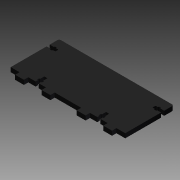
# Autodesk Inventor part: frontal base reforç
Saved by Autodesk Inventor 2012 SP1 (Build 160190100, 190)
## iProperties
Created: 2015-03-30
Part Number: frontal base reforç
Material: Default
Document SubType Name: Modeling
Designer: sheina
Density: 1 g/cm^3
Author: sheina
Autodesk Inventor part; units mm, degrees
ref_plane "YZ Plane" through (0, 0, 0) normal (1, 0, 0) x (0, 1, 0)
ref_plane "XZ Plane" through (0, 0, 0) normal (0, 1, 0) x (-1, 0, 0)
ref_plane "XY Plane" through (0, 0, 0) normal (0, 0, 1) x (1, 0, 0)
sketch "Boceto1" plane through (0, 0, 0) normal (0, 0, 1) x (1, 0, 0)
  line L0 (130, 10) -> (130, 65)
  line L1 (0, 65) -> (0, 10)
  line L2 (20, 10) -> (20, 5)
  line L3 (10, 5) -> (10, 10)
  line L4 (50, 10) -> (50, 5)
  line L5 (40, 5) -> (40, 10)
  line L6 (90, 10) -> (90, 5)
  line L7 (80, 5) -> (80, 10)
  line L8 (120, 10) -> (120, 5)
  line L9 (110, 5) -> (110, 10)
  line L10 (20, 5) -> (10, 5)
  line L11 (50, 5) -> (40, 5)
  line L12 (0, 10) -> (10, 10)
  line L13 (20, 10) -> (40, 10)
  line L14 (120, 5) -> (110, 5)
  line L15 (90, 5) -> (80, 5)
  line L16 (50, 10) -> (80, 10)
  line L17 (90, 10) -> (110, 10)
  line L18 (120, 10) -> (130, 10)
  line L19 (130, 65) -> (0, 65)
  point P0 (0, 0)
  dimension "d4" = 130
  dimension "d5" = 10
  dimension "d6" = 10
  dimension "d7" = 10
  dimension "d8" = 10
  dimension "d9" = 10
  dimension "d10" = 10
  dimension "d11" = 20
  dimension "d12" = 20
  dimension "d20" = 55
  constraints: 40 end point, 9 perpendicular, 6 parallel, 5 horizontal
  measures "d4" distance between parallel lines of L0 L1
  measures "d5" distance between parallel lines of L3 L2
  measures "d6" distance between parallel lines of L4 L5
  measures "d7" distance between parallel lines of L6 L7
  measures "d8" distance between parallel lines of L9 L8
  measures "d9" distance between parallel lines of L3 L1
  measures "d10" distance between parallel lines of L0 L8
  measures "d11" distance between parallel lines of L6 L9
  measures "d12" distance between parallel lines of L5 L2
  measures "d20" distance between parallel lines of L19 L13
extrude "Extrusión1" add sketch "Boceto1" along normal blind 5
fillet "Empalme1" radius 2 2 edges at (0, 65, 2.5) (130, 65, 2.5)
sketch "Boceto3" plane through (0, 0, 0) normal (0, 0, -1) x (-1, 0, 0)
  line L0 (-115.7878, 40.9736) -> (-8.9473, 40.9736) construction
  line L1 (-8.9473, 40.9736) -> (-8.9473, 10.5521) construction
  line L2 (-8.9473, 10.5521) -> (-115.7878, 10.5521) construction
  line L3 (-115.7878, 10.5521) -> (-115.7878, 40.9736) construction
  spline S0 degree 2 poles (-104.1512, 31.8359) (-104.5888, 31.8359) (-105.4543, 31.6219) (-105.8724, 31.4566) knots 0 0 0 1 2 2 2
  spline S1 degree 2 poles (-105.8724, 31.4566) (-106.2614, 31.2913) (-106.8351, 30.9412) (-107.0588, 30.7856) knots 0 0 0 1 2 2 2
  line L4 (-107.0588, 30.7856) -> (-107.156, 30.7856)
  line L5 (-107.156, 30.7856) -> (-107.156, 32.4874)
  spline S2 degree 2 poles (-107.156, 32.4874) (-106.6309, 32.7694) (-104.8319, 33.2265) (-104.0248, 33.2265) knots 0 0 0 1 2 2 2
  spline S3 degree 2 poles (-104.0248, 33.2265) (-103.2079, 33.2265) (-101.9923, 32.8958) (-101.4964, 32.5458) knots 0 0 0 1 2 2 2
  spline S4 degree 2 poles (-101.4964, 32.5458) (-100.9713, 32.1665) (-100.4267, 31.0676) (-100.4267, 30.3286) knots 0 0 0 1 2 2 2
  spline S5 degree 2 poles (-100.4267, 30.3286) (-100.4267, 29.3367) (-101.7298, 27.8391) (-102.6439, 27.6446) knots 0 0 0 1 2 2 2
  line L6 (-102.6439, 27.6446) -> (-102.6439, 27.5279)
  spline S6 degree 2 poles (-102.6439, 27.5279) (-102.2646, 27.4501) (-101.3992, 27.1001) (-101.0296, 26.75) knots 0 0 0 1 2 2 2
  spline S7 degree 2 poles (-101.0296, 26.75) (-100.6601, 26.4096) (-100.1933, 25.3205) (-100.1933, 24.5328) knots 0 0 0 1 2 2 2
  spline S8 degree 2 poles (-100.1933, 24.5328) (-100.1933, 23.7257) (-100.7476, 22.3545) (-101.2533, 21.8294) knots 0 0 0 1 2 2 2
  spline S9 degree 2 poles (-101.2533, 21.8294) (-101.7784, 21.2848) (-103.2663, 20.7208) (-104.2095, 20.7208) knots 0 0 0 1 2 2 2
  spline S10 degree 2 poles (-104.2095, 20.7208) (-105.1139, 20.7208) (-106.8838, 21.1584) (-107.4867, 21.4599) knots 0 0 0 1 2 2 2
  line L7 (-107.4867, 21.4599) -> (-107.4867, 23.1616)
  line L8 (-107.4867, 23.1616) -> (-107.37, 23.1616)
  spline S11 degree 2 poles (-107.37, 23.1616) (-106.8643, 22.7921) (-105.1528, 22.1114) (-104.3068, 22.1114) knots 0 0 0 1 2 2 2
  spline S12 degree 2 poles (-104.3068, 22.1114) (-103.8108, 22.1114) (-102.8189, 22.4226) (-102.4883, 22.7824) knots 0 0 0 1 2 2 2
  spline S13 degree 2 poles (-102.4883, 22.7824) (-102.1674, 23.1422) (-101.827, 23.9979) (-101.827, 24.6495) knots 0 0 0 1 2 2 2
  spline S14 degree 2 poles (-101.827, 24.6495) (-101.827, 25.301) (-102.2063, 26.1471) (-102.5466, 26.3902) knots 0 0 0 1 2 2 2
  spline S15 degree 2 poles (-102.5466, 26.3902) (-102.887, 26.6333) (-103.8108, 26.818) (-104.3554, 26.818) knots 0 0 0 1 2 2 2
  line L9 (-104.3554, 26.818) -> (-105.0361, 26.818)
  line L10 (-105.0361, 26.818) -> (-105.0361, 28.1503)
  line L11 (-105.0361, 28.1503) -> (-104.5013, 28.1503)
  spline S16 degree 2 poles (-104.5013, 28.1503) (-103.4218, 28.1503) (-102.0604, 29.1811) (-102.0604, 30.1633) knots 0 0 0 1 2 2 2
  spline S17 degree 2 poles (-102.0604, 30.1633) (-102.0604, 30.6203) (-102.4105, 31.2719) (-102.6925, 31.4663) knots 0 0 0 1 2 2 2
  spline S18 degree 2 poles (-102.6925, 31.4663) (-102.994, 31.6706) (-103.733, 31.8359) (-104.1512, 31.8359) knots 0 0 0 1 2 2 2
  spline S19 degree 2 poles (-88.5823, 26.9639) (-88.5823, 25.3205) (-89.9146, 22.6754) (-91.0329, 21.9364) knots 0 0 0 1 2 2 2
  spline S20 degree 2 poles (-91.0329, 21.9364) (-91.947, 21.3626) (-93.8238, 20.9736) (-95.2825, 20.9736) knots 0 0 0 1 2 2 2
  line L12 (-95.2825, 20.9736) -> (-98.0442, 20.9736)
  line L13 (-98.0442, 20.9736) -> (-98.0442, 32.9736)
  line L14 (-98.0442, 32.9736) -> (-95.3116, 32.9736)
  spline S21 degree 2 poles (-95.3116, 32.9736) (-93.6196, 32.9736) (-91.6941, 32.468) (-91.0134, 32.0206) knots 0 0 0 1 2 2 2
  spline S22 degree 2 poles (-91.0134, 32.0206) (-89.8562, 31.2524) (-88.5823, 28.7143) (-88.5823, 26.9639) knots 0 0 0 1 2 2 2
  spline S23 degree 2 poles (-90.2452, 26.9834) (-90.2452, 28.3642) (-91.1593, 30.3189) (-92.0637, 30.8731) knots 0 0 0 1 2 2 2
  spline S24 degree 2 poles (-92.0637, 30.8731) (-92.7055, 31.2524) (-94.1544, 31.5928) (-95.2338, 31.5928) knots 0 0 0 1 2 2 2
  line L15 (-95.2338, 31.5928) -> (-96.4494, 31.5928)
  line L16 (-96.4494, 31.5928) -> (-96.4494, 22.3545)
  line L17 (-96.4494, 22.3545) -> (-95.2338, 22.3545)
  spline S25 degree 2 poles (-95.2338, 22.3545) (-94.1739, 22.3545) (-92.5693, 22.6949) (-91.9178, 23.1519) knots 0 0 0 1 2 2 2
  spline S26 degree 2 poles (-91.9178, 23.1519) (-91.0815, 23.7159) (-90.2452, 25.583) (-90.2452, 26.9834) knots 0 0 0 1 2 2 2
  spline S27 degree 2 poles (-72.1431, 27.959) (-72.1431, 27.3107) (-72.605, 26.1438) (-73.0183, 25.7386) knots 0 0 0 1 2 2 2
  spline S28 degree 2 poles (-73.0183, 25.7386) (-73.5369, 25.2281) (-74.9389, 24.7013) (-76.0086, 24.7013) knots 0 0 0 1 2 2 2
  line L18 (-76.0086, 24.7013) -> (-77.135, 24.7013)
  line L19 (-77.135, 24.7013) -> (-77.135, 20.9736)
  line L20 (-77.135, 20.9736) -> (-78.464, 20.9736)
  line L21 (-78.464, 20.9736) -> (-78.464, 30.9736)
  line L22 (-78.464, 30.9736) -> (-75.9518, 30.9736)
  spline S29 degree 2 poles (-75.9518, 30.9736) (-75.0604, 30.9736) (-73.8124, 30.6819) (-73.3343, 30.3496) knots 0 0 0 1 2 2 2
  spline S30 degree 2 poles (-73.3343, 30.3496) (-72.7752, 29.9688) (-72.1431, 28.7937) (-72.1431, 27.959) knots 0 0 0 1 2 2 2
  spline S31 degree 2 poles (-73.5288, 27.9185) (-73.5288, 28.4372) (-73.8854, 29.1989) (-74.25, 29.442) knots 0 0 0 1 2 2 2
  spline S32 degree 2 poles (-74.25, 29.442) (-74.5661, 29.6527) (-75.4089, 29.8229) (-76.0329, 29.8229) knots 0 0 0 1 2 2 2
  line L23 (-76.0329, 29.8229) -> (-77.135, 29.8229)
  line L24 (-77.135, 29.8229) -> (-77.135, 25.8359)
  line L25 (-77.135, 25.8359) -> (-76.2274, 25.8359)
  spline S33 degree 2 poles (-76.2274, 25.8359) (-75.417, 25.8359) (-74.4202, 26.0952) (-74.0961, 26.4355) knots 0 0 0 1 2 2 2
  spline S34 degree 2 poles (-74.0961, 26.4355) (-73.7962, 26.7354) (-73.5288, 27.4404) (-73.5288, 27.9185) knots 0 0 0 1 2 2 2
  line L26 (-63.1398, 20.9736) -> (-64.8659, 20.9736)
  line L27 (-64.8659, 20.9736) -> (-68.0264, 24.9526)
  line L28 (-68.0264, 24.9526) -> (-69.5499, 24.9526)
  line L29 (-69.5499, 24.9526) -> (-69.5499, 20.9736)
  line L30 (-69.5499, 20.9736) -> (-70.8789, 20.9736)
  line L31 (-70.8789, 20.9736) -> (-70.8789, 30.9736)
  line L32 (-70.8789, 30.9736) -> (-68.3019, 30.9736)
  spline S35 degree 2 poles (-68.3019, 30.9736) (-67.4429, 30.9736) (-66.2841, 30.7872) (-65.7573, 30.4469) knots 0 0 0 1 2 2 2
  spline S36 degree 2 poles (-65.7573, 30.4469) (-65.2306, 30.1065) (-64.6228, 29.0449) (-64.6228, 28.2589) knots 0 0 0 1 2 2 2
  spline S37 degree 2 poles (-64.6228, 28.2589) (-64.6228, 27.1649) (-65.7411, 25.6819) (-66.6974, 25.3253) knots 0 0 0 1 2 2 2
  line L33 (-66.6974, 25.3253) -> (-63.1398, 20.9736)
  spline S38 degree 2 poles (-66.0086, 28.1535) (-66.0086, 28.5911) (-66.3165, 29.2637) (-66.6406, 29.4825) knots 0 0 0 1 2 2 2
  spline S39 degree 2 poles (-66.6406, 29.4825) (-66.9243, 29.6689) (-67.6779, 29.8229) (-68.229, 29.8229) knots 0 0 0 1 2 2 2
  line L34 (-68.229, 29.8229) -> (-69.5499, 29.8229)
  line L35 (-69.5499, 29.8229) -> (-69.5499, 26.0628)
  line L36 (-69.5499, 26.0628) -> (-68.3829, 26.0628)
  spline S40 degree 2 poles (-68.3829, 26.0628) (-67.8076, 26.0628) (-66.8919, 26.2654) (-66.5758, 26.5814) knots 0 0 0 1 2 2 2
  spline S41 degree 2 poles (-66.5758, 26.5814) (-66.2841, 26.8569) (-66.0086, 27.6349) (-66.0086, 28.1535) knots 0 0 0 1 2 2 2
  line L37 (-58.8611, 20.9736) -> (-62.7346, 20.9736)
  line L38 (-62.7346, 20.9736) -> (-62.7346, 21.9947)
  line L39 (-62.7346, 21.9947) -> (-61.4624, 21.9947)
  line L40 (-61.4624, 21.9947) -> (-61.4624, 29.9526)
  line L41 (-61.4624, 29.9526) -> (-62.7346, 29.9526)
  line L42 (-62.7346, 29.9526) -> (-62.7346, 30.9736)
  line L43 (-62.7346, 30.9736) -> (-58.8611, 30.9736)
  line L44 (-58.8611, 30.9736) -> (-58.8611, 29.9526)
  line L45 (-58.8611, 29.9526) -> (-60.1334, 29.9526)
  line L46 (-60.1334, 29.9526) -> (-60.1334, 21.9947)
  line L47 (-60.1334, 21.9947) -> (-58.8611, 21.9947)
  line L48 (-58.8611, 21.9947) -> (-58.8611, 20.9736)
  line L49 (-50.0604, 20.9736) -> (-51.5515, 20.9736)
  line L50 (-51.5515, 20.9736) -> (-55.9761, 29.596)
  line L51 (-55.9761, 29.596) -> (-55.9761, 20.9736)
  line L52 (-55.9761, 20.9736) -> (-57.216, 20.9736)
  line L53 (-57.216, 20.9736) -> (-57.216, 30.9736)
  line L54 (-57.216, 30.9736) -> (-55.3278, 30.9736)
  line L55 (-55.3278, 30.9736) -> (-51.3003, 23.0563)
  line L56 (-51.3003, 23.0563) -> (-51.3003, 30.9736)
  line L57 (-51.3003, 30.9736) -> (-50.0604, 30.9736)
  line L58 (-50.0604, 30.9736) -> (-50.0604, 20.9736)
  line L59 (-45.7006, 20.9736) -> (-45.7006, 29.7905)
  line L60 (-45.7006, 29.7905) -> (-49.0556, 29.7905)
  line L61 (-49.0556, 29.7905) -> (-49.0556, 30.9736)
  line L62 (-49.0556, 30.9736) -> (-41.0167, 30.9736)
  line L63 (-41.0167, 30.9736) -> (-41.0167, 29.7905)
  line L64 (-41.0167, 29.7905) -> (-44.3716, 29.7905)
  line L65 (-44.3716, 29.7905) -> (-44.3716, 20.9736)
  line L66 (-44.3716, 20.9736) -> (-45.7006, 20.9736)
  spline S42 degree 2 poles (-36.0977, 20.7954) (-37.0701, 20.7954) (-38.7152, 21.4518) (-39.3149, 22.1082) knots 0 0 0 1 2 2 2
  spline S43 degree 2 poles (-39.3149, 22.1082) (-39.9145, 22.7565) (-40.571, 24.7013) (-40.571, 25.9655) knots 0 0 0 1 2 2 2
  spline S44 degree 2 poles (-40.571, 25.9655) (-40.571, 27.2216) (-39.9308, 29.0855) (-39.323, 29.7743) knots 0 0 0 1 2 2 2
  spline S45 degree 2 poles (-39.323, 29.7743) (-38.7233, 30.4469) (-37.0863, 31.1519) (-36.0734, 31.1519) knots 0 0 0 1 2 2 2
  spline S46 degree 2 poles (-36.0734, 31.1519) (-35.571, 31.1519) (-34.6876, 31.006) (-34.3149, 30.8926) knots 0 0 0 1 2 2 2
  spline S47 degree 2 poles (-34.3149, 30.8926) (-33.9907, 30.7872) (-33.3181, 30.4874) (-32.9859, 30.3091) knots 0 0 0 1 2 2 2
  line L67 (-32.9859, 30.3091) -> (-32.9859, 28.7046)
  line L68 (-32.9859, 28.7046) -> (-33.0912, 28.7046)
  spline S48 degree 2 poles (-33.0912, 28.7046) (-33.2695, 28.8667) (-33.8205, 29.3205) (-34.2176, 29.5393) knots 0 0 0 1 2 2 2
  spline S49 degree 2 poles (-34.2176, 29.5393) (-34.5985, 29.75) (-35.498, 30.0174) (-36.0815, 30.0174) knots 0 0 0 1 2 2 2
  spline S50 degree 2 poles (-36.0815, 30.0174) (-36.7217, 30.0174) (-37.8643, 29.4907) (-38.2938, 28.9882) knots 0 0 0 1 2 2 2
  spline S51 degree 2 poles (-38.2938, 28.9882) (-38.7152, 28.4777) (-39.1852, 26.9299) (-39.1852, 25.9655) knots 0 0 0 1 2 2 2
  spline S52 degree 2 poles (-39.1852, 25.9655) (-39.1852, 24.9364) (-38.6909, 23.4534) (-38.2614, 22.9428) knots 0 0 0 1 2 2 2
  spline S53 degree 2 poles (-38.2614, 22.9428) (-37.84, 22.4485) (-36.7136, 21.9461) (-36.0815, 21.9461) knots 0 0 0 1 2 2 2
  spline S54 degree 2 poles (-36.0815, 21.9461) (-35.5061, 21.9461) (-34.5256, 22.2297) (-34.1447, 22.4404) knots 0 0 0 1 2 2 2
  spline S55 degree 2 poles (-34.1447, 22.4404) (-33.78, 22.6511) (-33.2371, 23.0887) (-33.0831, 23.2427) knots 0 0 0 1 2 2 2
  line L69 (-33.0831, 23.2427) -> (-32.9859, 23.2427)
  line L70 (-32.9859, 23.2427) -> (-32.9859, 21.6543)
  spline S56 degree 2 poles (-32.9859, 21.6543) (-33.3181, 21.5004) (-33.9016, 21.2167) (-34.3149, 21.0871) knots 0 0 0 1 2 2 2
  spline S57 degree 2 poles (-34.3149, 21.0871) (-34.7525, 20.9412) (-35.498, 20.7954) (-36.0977, 20.7954) knots 0 0 0 1 2 2 2
  line L71 (-32.8238, 20.9736) -> (-29.4526, 30.9736)
  line L72 (-29.4526, 30.9736) -> (-27.8157, 30.9736)
  line L73 (-27.8157, 30.9736) -> (-24.4445, 20.9736)
  line L74 (-24.4445, 20.9736) -> (-25.8465, 20.9736)
  line L75 (-25.8465, 20.9736) -> (-26.7541, 23.7694)
  line L76 (-26.7541, 23.7694) -> (-30.571, 23.7694)
  line L77 (-30.571, 23.7694) -> (-31.4786, 20.9736)
  line L78 (-31.4786, 20.9736) -> (-32.8238, 20.9736)
  line L79 (-27.1188, 24.9039) -> (-28.6666, 29.6122)
  line L80 (-28.6666, 29.6122) -> (-30.2063, 24.9039)
  line L81 (-30.2063, 24.9039) -> (-27.1188, 24.9039)
  line L82 (-21.1625, 20.9736) -> (-21.1625, 29.7905)
  line L83 (-21.1625, 29.7905) -> (-24.5175, 29.7905)
  line L84 (-24.5175, 29.7905) -> (-24.5175, 30.9736)
  line L85 (-24.5175, 30.9736) -> (-16.4786, 30.9736)
  line L86 (-16.4786, 30.9736) -> (-16.4786, 29.7905)
  line L87 (-16.4786, 29.7905) -> (-19.8335, 29.7905)
  line L88 (-19.8335, 29.7905) -> (-19.8335, 20.9736)
  line L89 (-19.8335, 20.9736) -> (-21.1625, 20.9736)
  constraints: 2 other
extrude "Extrusión3" cut sketch "Boceto3" against normal blind 1
sketch "Boceto4" plane through (0, 0, 0) normal (0, 0, -1) x (-1, 0, 0)
  line L0 (-31.7524, 12.5727) -> (-32.7524, 12.5727)
  line L1 (-31.7524, 9.7986) -> (-31.7524, 12.5727)
  line L2 (-31.7524, 14.9727) -> (-31.7524, 19.884)
  line L3 (-27.2524, 14.9727) -> (-27.2524, 12.5727)
  line L4 (-28.2524, 14.9727) -> (-27.2524, 14.9727)
  line L5 (-31.7524, 19.884) -> (-28.2524, 19.884)
  line L6 (-28.2524, 19.884) -> (-28.2524, 14.9727)
  line L7 (-27.2524, 12.5727) -> (-28.2524, 12.5727)
  line L8 (-28.2524, 12.5727) -> (-28.2524, 9.7986)
  line L9 (-32.7524, 12.5727) -> (-32.7524, 14.9727)
  line L10 (-32.7524, 14.9727) -> (-31.7524, 14.9727)
  line L11 (-31.7524, 9.7986) -> (-28.2524, 9.7986)
  line L12 (-101.7513, 12.6989) -> (-102.7513, 12.6989)
  line L13 (-101.7513, 9.9249) -> (-101.7513, 12.6989)
  line L14 (-101.7513, 15.0989) -> (-101.7513, 20.0103)
  line L15 (-97.2513, 15.0989) -> (-97.2513, 12.6989)
  line L16 (-98.2513, 15.0989) -> (-97.2513, 15.0989)
  line L17 (-101.7513, 20.0103) -> (-98.2513, 20.0103)
  line L18 (-98.2513, 20.0103) -> (-98.2513, 15.0989)
  line L19 (-97.2513, 12.6989) -> (-98.2513, 12.6989)
  line L20 (-98.2513, 12.6989) -> (-98.2513, 9.9249)
  line L21 (-102.7513, 12.6989) -> (-102.7513, 15.0989)
  line L22 (-102.7513, 15.0989) -> (-101.7513, 15.0989)
  line L23 (-101.7513, 9.9249) -> (-98.2513, 9.9249)
  line L24 (-123.0301, 50.7481) -> (-123.0301, 49.7481)
  line L25 (-120.2561, 50.7481) -> (-123.0301, 50.7481)
  line L26 (-125.4301, 50.7481) -> (-130.3414, 50.7481)
  line L27 (-125.4301, 55.2481) -> (-123.0301, 55.2481)
  line L28 (-125.4301, 54.2481) -> (-125.4301, 55.2481)
  line L29 (-130.3414, 50.7481) -> (-130.3414, 54.2481)
  line L30 (-130.3414, 54.2481) -> (-125.4301, 54.2481)
  line L31 (-123.0301, 55.2481) -> (-123.0301, 54.2481)
  line L32 (-123.0301, 54.2481) -> (-120.2561, 54.2481)
  line L33 (-123.0301, 49.7481) -> (-125.4301, 49.7481)
  line L34 (-125.4301, 49.7481) -> (-125.4301, 50.7481)
  line L35 (-120.2561, 50.7481) -> (-120.2561, 54.2481)
  line L36 (0.1688, 50.7361) -> (-4.7425, 50.7361)
  line L37 (0.1688, 54.2361) -> (0.1688, 50.7361)
  line L38 (-4.7425, 54.2361) -> (0.1688, 54.2361)
  line L39 (-4.7425, 50.7361) -> (-4.7425, 49.7361)
  line L40 (-7.1425, 49.7361) -> (-7.1425, 50.7361)
  line L41 (-7.1425, 50.7361) -> (-9.9165, 50.7361)
  line L42 (-9.9165, 54.2361) -> (-7.1425, 54.2361)
  line L43 (-4.7425, 55.2361) -> (-4.7425, 54.2361)
  line L44 (-7.1425, 55.2361) -> (-4.7425, 55.2361)
  line L45 (-7.1425, 54.2361) -> (-7.1425, 55.2361)
  line L46 (-9.9165, 54.2361) -> (-9.9165, 50.7361)
  line L47 (-4.7425, 49.7361) -> (-7.1425, 49.7361)
  point P0 (0, 0)
  dimension "d21" = 3.5
  dimension "d22" = 3.5
  dimension "d23" = 3.5
  dimension "d24" = 3.5
  constraints: 96 end point
  measures "d21" distance between parallel lines of L8 L1
  measures "d22" distance between parallel lines of L20 L13
  measures "d23" distance between parallel lines of L32 L25
  measures "d24" distance between parallel lines of L41 L42
extrude "Extrusión4" cut sketch "Boceto4" against normal blind 10
equation "\"d6\" = d5"
equation "\"d7\" = d5"
equation "\"d8\" = d5"
